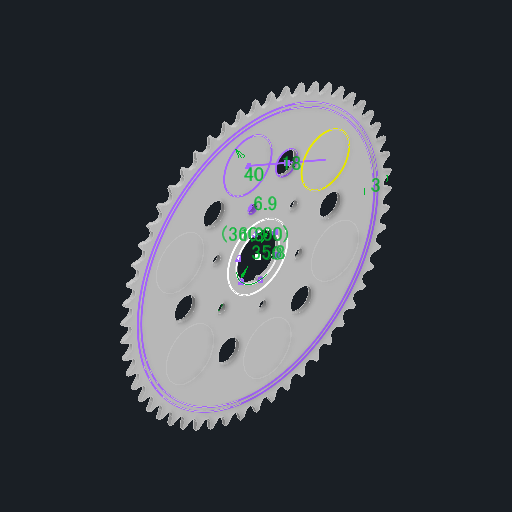
# Autodesk Inventor part: 410A54_()
Saved by Autodesk Inventor 2025.2 (Build 292293000, 293)
## iProperties
Category: PARTsolutions
Company: KANA
Created: 2025-03-16
Part Number: 410A54_()
Material: Generic
Catalog Web Link: www.cadenas.de
Description: 410A-Un-finished
Vendor: KANA
Document SubType Name: Modeling
Designer: psAdmin
Manufacturer: KANA
Mass: 102.167 g
Surface Area: 762.68 cm^2
Volume: 102.167 cm^3
Density: 1 g/cm^3
Appearance: PSOLRGB-175-175-175
PSOL_IDENT_0: {$CADENAS_DATA/23d-libs/kana/sprockets/chain_no_410/un_finished_sprocket_steel/a_type/410a.prj},159
PSOL_IDENT_1: {VTYP=3D},{NB=410A54_()},{LINA=410A54},{NN=410A},{DATE=27.06.2023 01:46:24},{GEOMDATE=02.10.2020 05:
PSOL_IDENT_2: 05:48},{VERSION=},{LINEID=690},{WBVAR=SURFT},{WBNUMERIC=}  {NB=410A54_()},{LINA=410A54},{KT=DUMMY},{
PSOL_IDENT_3: ORDERNO=410A54},{TYPE=410A},{NOT=54},{NOTX=54.000},{DP=218.42},{DC=210.67},{DC2=210.67},{DO=226},{T=
PSOL_IDENT_4: 2.8},{DR=7.750},{MAT=None},{MATC=},{SD=16},{SURFT=},{SURFTNB=},{DCX2=0},{CAUTION=The tooth profile i
PSOL_IDENT_5: n the CAD models differ from the actual shape.}
NB: 410A54_()
NN: 410A
NT: Un-finished
NBSYN: 410A$NOT._($SURFT.)
LINA: 410A54
CATALOG: KANA
TYPE: 410A
NOT: 54
DP: 218.42
DC: 210.67
DC2: 210.67
DO: 226
T: 2.8
SD: 16
SURFT: No symbol : No
CAUTION: The tooth profile in the CAD models differ from the actual shape.
SUPPLIER: KANA
ARTICLENO: 410A54_()
BOMINFO: 410A54
CREATOR: CADENAS GmbH
Title: 410A54
Author: Cadenas PARTsolutions
Comments: Un-finished
Autodesk Inventor part; units mm, degrees
sketch "Sketch_1" plane through (0, 0, 0) normal (0, 0, 1) x (1, 0, 0)
  line L0 (2.8, 0) -> (0, 0)
  line L1 (0, 8) -> (2.8, 8)
  line L2 (2.8, 8) -> (2.8, 111.7584)
  arc A0 (2.8, 111.7584) -> (2.1, 113) centre (-4.2724, 108.5892) ccw
  line L3 (2.1, 113) -> (0.7, 113)
  arc A1 (0.7, 113) -> (0, 111.7584) centre (7.0724, 108.5892) ccw
  line L4 (0, 111.7584) -> (0, 8)
  constraints: 10 end point, 4 point on circle, 2 centre point
revolve "Revolution1" add sketch "Sketch_1" angle 360 about axis through (2.8, 0, 0) along (1, 0, 0)
sketch "Sketch_2" plane through (1.4, 0, 0) normal (1, 0, 0) x (0, 0, -1)
  circle A0 centre (0, 0) radius 150.6667
  line L0 (-112.8368, 6.0711) -> (-107.5161, 3.4852)
  arc A1 (-107.5161, -3.4852) -> (-107.5161, 3.4852) centre (-109.21, 0) ccw
  line L1 (-107.5161, -3.4852) -> (-112.8368, -6.0711)
  arc A2 (-112.8368, -6.0711) -> (-112.7786, -7.0695) centre (0, 0) ccw
  line L2 (-112.7786, -7.0695) -> (-107.1937, -9.0203)
  arc A3 (-106.3845, -15.9435) -> (-107.1937, -9.0203) centre (-108.4716, -12.6785) ccw
  line L3 (-106.3845, -15.9435) -> (-111.369, -19.1296)
  arc A4 (-111.369, -19.1296) -> (-111.1954, -20.1145) centre (0, 0) ccw
  line L4 (-111.1954, -20.1145) -> (-105.4217, -21.4037)
  arc A5 (-103.8143, -28.1861) -> (-105.4217, -21.4037) centre (-106.2662, -25.1856) ccw
  line L5 (-103.8143, -28.1861) -> (-108.3952, -31.9295)
  arc A6 (-108.3952, -31.9295) -> (-108.1084, -32.8874) centre (0, 0) ccw
  line L6 (-108.1084, -32.8874) -> (-102.2241, -33.4977)
  arc A7 (-99.8401, -40.0477) -> (-102.2241, -33.4977) centre (-102.6238, -37.352) ccw
  line L7 (-99.8401, -40.0477) -> (-103.9554, -44.2975)
  arc A8 (-103.9554, -44.2975) -> (-103.5594, -45.2157) centre (0, 0) ccw
  line L8 (-103.5594, -45.2157) -> (-97.6441, -45.1387)
  arc A9 (-94.5158, -51.3676) -> (-97.6441, -45.1387) centre (-97.5936, -49.0134) ccw
  line L9 (-94.5158, -51.3676) -> (-98.1099, -56.0664)
  arc A10 (-98.1099, -56.0664) -> (-97.6099, -56.9325) centre (0, 0) ccw
  line L10 (-97.6099, -56.9325) -> (-91.7435, -56.1693)
  arc A11 (-87.9133, -61.9929) -> (-91.7435, -56.1693) centre (-91.2436, -60.0119) ccw
  line L11 (-87.9133, -61.9929) -> (-90.9376, -67.0772)
  arc A12 (-90.9376, -67.0772) -> (-90.3405, -67.8793) centre (0, 0) ccw
  line L12 (-90.3405, -67.8793) -> (-84.6023, -66.4402)
  arc A13 (-80.1219, -71.7798) -> (-84.6023, -66.4402) centre (-83.6597, -70.1988) ccw
  line L13 (-80.1219, -71.7798) -> (-82.5355, -77.1809)
  arc A14 (-82.5355, -77.1809) -> (-81.8493, -77.9082) centre (0, 0) ccw
  line L14 (-81.8493, -77.9082) -> (-76.3171, -75.8127)
  arc A15 (-71.247, -80.5961) -> (-76.3171, -75.8127) centre (-74.9444, -79.4365) ccw
  line L15 (-71.247, -80.5961) -> (-73.0173, -86.2408)
  arc A16 (-73.0173, -86.2408) -> (-72.2513, -86.8836) centre (0, 0) ccw
  line L16 (-72.2513, -86.8836) -> (-66.9997, -84.16)
  arc A17 (-61.4086, -88.3224) -> (-66.9997, -84.16) centre (-65.2157, -87.5999) ccw
  line L17 (-61.4086, -88.3224) -> (-62.5117, -94.1344)
  arc A18 (-62.5117, -94.1344) -> (-61.6762, -94.684) centre (0, 0) ccw
  line L18 (-61.6762, -94.684) -> (-56.7763, -91.3691)
  arc A19 (-50.7398, -94.8543) -> (-56.7763, -91.3691) centre (-54.605, -94.5786) ccw
  line L19 (-50.7398, -94.8543) -> (-51.1606, -100.7551)
  arc A20 (-51.1606, -100.7551) -> (-50.267, -101.2039) centre (0, 0) ccw
  line L20 (-50.267, -101.2039) -> (-45.7851, -97.3426)
  arc A21 (-39.3848, -100.1034) -> (-45.7851, -97.3426) centre (-43.2559, -100.2784) ccw
  line L21 (-39.3848, -100.1034) -> (-39.1177, -106.0132)
  arc A22 (-39.1177, -106.0132) -> (-38.1781, -106.3552) centre (0, 0) ccw
  line L22 (-38.1781, -106.3552) -> (-34.1747, -101.9998)
  arc A23 (-27.4972, -103.9989) -> (-34.1747, -101.9998) centre (-31.3218, -104.622) ccw
  line L23 (-27.4972, -103.9989) -> (-26.5459, -109.8377)
  arc A24 (-26.5459, -109.8377) -> (-25.5728, -110.0683) centre (0, 0) ccw
  line L24 (-25.5728, -110.0683) -> (-22.1022, -105.2775)
  arc A25 (-15.2378, -106.4879) -> (-22.1022, -105.2775) centre (-18.9641, -107.5509) ccw
  line L25 (-15.2378, -106.4879) -> (-13.615, -112.1768)
  arc A26 (-13.615, -112.1768) -> (-12.6218, -112.2929) centre (0, 0) ccw
  line L26 (-12.6218, -112.2929) -> (-9.7308, -107.1316)
  arc A27 (-2.7722, -107.5369) -> (-9.7308, -107.1316) centre (-6.35, -109.0252) ccw
  line L27 (-2.7722, -107.5369) -> (-0.5, -112.9989)
  arc A28 (-0.5, -112.9989) -> (0.5, -112.9989) centre (0, 0) ccw
  line L28 (0.5, -112.9989) -> (2.7722, -107.5369)
  arc A29 (9.7308, -107.1316) -> (2.7722, -107.5369) centre (6.35, -109.0252) ccw
  line L29 (9.7308, -107.1316) -> (12.6218, -112.2929)
  arc A30 (12.6218, -112.2929) -> (13.615, -112.1768) centre (0, 0) ccw
  line L30 (13.615, -112.1768) -> (15.2378, -106.4879)
  arc A31 (22.1022, -105.2775) -> (15.2378, -106.4879) centre (18.9641, -107.5509) ccw
  line L31 (22.1022, -105.2775) -> (25.5728, -110.0683)
  arc A32 (25.5728, -110.0683) -> (26.5459, -109.8377) centre (0, 0) ccw
  line L32 (26.5459, -109.8377) -> (27.4972, -103.9989)
  arc A33 (34.1747, -101.9998) -> (27.4972, -103.9989) centre (31.3218, -104.622) ccw
  line L33 (34.1747, -101.9998) -> (38.1781, -106.3552)
  arc A34 (38.1781, -106.3552) -> (39.1177, -106.0132) centre (0, 0) ccw
  line L34 (39.1177, -106.0132) -> (39.3848, -100.1034)
  arc A35 (45.7851, -97.3426) -> (39.3848, -100.1034) centre (43.2559, -100.2784) ccw
  line L35 (45.7851, -97.3426) -> (50.267, -101.2039)
  arc A36 (50.267, -101.2039) -> (51.1606, -100.7551) centre (0, 0) ccw
  line L36 (51.1606, -100.7551) -> (50.7398, -94.8543)
  arc A37 (56.7763, -91.3691) -> (50.7398, -94.8543) centre (54.605, -94.5786) ccw
  line L37 (56.7763, -91.3691) -> (61.6762, -94.684)
  arc A38 (61.6762, -94.684) -> (62.5117, -94.1344) centre (0, 0) ccw
  line L38 (62.5117, -94.1344) -> (61.4086, -88.3224)
  arc A39 (66.9997, -84.16) -> (61.4086, -88.3224) centre (65.2157, -87.5999) ccw
  line L39 (66.9997, -84.16) -> (72.2513, -86.8836)
  arc A40 (72.2513, -86.8836) -> (73.0173, -86.2408) centre (0, 0) ccw
  line L40 (73.0173, -86.2408) -> (71.247, -80.5961)
  arc A41 (76.3171, -75.8127) -> (71.247, -80.5961) centre (74.9444, -79.4365) ccw
  line L41 (76.3171, -75.8127) -> (81.8493, -77.9082)
  arc A42 (81.8493, -77.9082) -> (82.5355, -77.1809) centre (0, 0) ccw
  line L42 (82.5355, -77.1809) -> (80.1219, -71.7798)
  arc A43 (84.6023, -66.4402) -> (80.1219, -71.7798) centre (83.6597, -70.1988) ccw
  line L43 (84.6023, -66.4402) -> (90.3405, -67.8793)
  arc A44 (90.3405, -67.8793) -> (90.9376, -67.0772) centre (0, 0) ccw
  line L44 (90.9376, -67.0772) -> (87.9133, -61.9929)
  arc A45 (91.7435, -56.1693) -> (87.9133, -61.9929) centre (91.2436, -60.0119) ccw
  line L45 (91.7435, -56.1693) -> (97.6099, -56.9325)
  arc A46 (97.6099, -56.9325) -> (98.1099, -56.0664) centre (0, 0) ccw
  line L46 (98.1099, -56.0664) -> (94.5158, -51.3676)
  arc A47 (97.6441, -45.1387) -> (94.5158, -51.3676) centre (97.5936, -49.0134) ccw
  line L47 (97.6441, -45.1387) -> (103.5594, -45.2157)
  arc A48 (103.5594, -45.2157) -> (103.9554, -44.2975) centre (0, 0) ccw
  line L48 (103.9554, -44.2975) -> (99.8401, -40.0477)
  arc A49 (102.2241, -33.4977) -> (99.8401, -40.0477) centre (102.6238, -37.352) ccw
  line L49 (102.2241, -33.4977) -> (108.1084, -32.8874)
  arc A50 (108.1084, -32.8874) -> (108.3952, -31.9295) centre (0, 0) ccw
  line L50 (108.3952, -31.9295) -> (103.8143, -28.1861)
  arc A51 (105.4217, -21.4037) -> (103.8143, -28.1861) centre (106.2662, -25.1856) ccw
  line L51 (105.4217, -21.4037) -> (111.1954, -20.1145)
  arc A52 (111.1954, -20.1145) -> (111.369, -19.1296) centre (0, 0) ccw
  line L52 (111.369, -19.1296) -> (106.3845, -15.9435)
  arc A53 (107.1937, -9.0203) -> (106.3845, -15.9435) centre (108.4716, -12.6785) ccw
  line L53 (107.1937, -9.0203) -> (112.7786, -7.0695)
  arc A54 (112.7786, -7.0695) -> (112.8368, -6.0711) centre (0, 0) ccw
  line L54 (112.8368, -6.0711) -> (107.5161, -3.4852)
  arc A55 (107.5161, 3.4852) -> (107.5161, -3.4852) centre (109.21, 0) ccw
  line L55 (107.5161, 3.4852) -> (112.8368, 6.0711)
  arc A56 (112.8368, 6.0711) -> (112.7786, 7.0695) centre (0, 0) ccw
  line L56 (112.7786, 7.0695) -> (107.1937, 9.0203)
  arc A57 (106.3845, 15.9435) -> (107.1937, 9.0203) centre (108.4716, 12.6785) ccw
  line L57 (106.3845, 15.9435) -> (111.369, 19.1296)
  arc A58 (111.369, 19.1296) -> (111.1954, 20.1145) centre (0, 0) ccw
  line L58 (111.1954, 20.1145) -> (105.4217, 21.4037)
  arc A59 (103.8143, 28.1861) -> (105.4217, 21.4037) centre (106.2662, 25.1856) ccw
  line L59 (103.8143, 28.1861) -> (108.3952, 31.9295)
  arc A60 (108.3952, 31.9295) -> (108.1084, 32.8874) centre (0, 0) ccw
  line L60 (108.1084, 32.8874) -> (102.2241, 33.4977)
  arc A61 (99.8401, 40.0477) -> (102.2241, 33.4977) centre (102.6238, 37.352) ccw
  line L61 (99.8401, 40.0477) -> (103.9554, 44.2975)
  arc A62 (103.9554, 44.2975) -> (103.5594, 45.2157) centre (0, 0) ccw
  line L62 (103.5594, 45.2157) -> (97.6441, 45.1387)
  arc A63 (94.5158, 51.3676) -> (97.6441, 45.1387) centre (97.5936, 49.0134) ccw
  line L63 (94.5158, 51.3676) -> (98.1099, 56.0664)
  arc A64 (98.1099, 56.0664) -> (97.6099, 56.9325) centre (0, 0) ccw
  line L64 (97.6099, 56.9325) -> (91.7435, 56.1693)
  arc A65 (87.9133, 61.9929) -> (91.7435, 56.1693) centre (91.2436, 60.0119) ccw
  line L65 (87.9133, 61.9929) -> (90.9376, 67.0772)
  arc A66 (90.9376, 67.0772) -> (90.3405, 67.8793) centre (0, 0) ccw
  line L66 (90.3405, 67.8793) -> (84.6023, 66.4402)
  arc A67 (80.1219, 71.7798) -> (84.6023, 66.4402) centre (83.6597, 70.1988) ccw
  line L67 (80.1219, 71.7798) -> (82.5355, 77.1809)
  arc A68 (82.5355, 77.1809) -> (81.8493, 77.9082) centre (0, 0) ccw
  line L68 (81.8493, 77.9082) -> (76.3171, 75.8127)
  arc A69 (71.247, 80.5961) -> (76.3171, 75.8127) centre (74.9444, 79.4365) ccw
  line L69 (71.247, 80.5961) -> (73.0173, 86.2408)
  arc A70 (73.0173, 86.2408) -> (72.2513, 86.8836) centre (0, 0) ccw
  line L70 (72.2513, 86.8836) -> (66.9997, 84.16)
  arc A71 (61.4086, 88.3224) -> (66.9997, 84.16) centre (65.2157, 87.5999) ccw
  line L71 (61.4086, 88.3224) -> (62.5117, 94.1344)
  arc A72 (62.5117, 94.1344) -> (61.6762, 94.684) centre (0, 0) ccw
  line L72 (61.6762, 94.684) -> (56.7763, 91.3691)
  arc A73 (50.7398, 94.8543) -> (56.7763, 91.3691) centre (54.605, 94.5786) ccw
  line L73 (50.7398, 94.8543) -> (51.1606, 100.7551)
  arc A74 (51.1606, 100.7551) -> (50.267, 101.2039) centre (0, 0) ccw
  line L74 (50.267, 101.2039) -> (45.7851, 97.3426)
  arc A75 (39.3848, 100.1034) -> (45.7851, 97.3426) centre (43.2559, 100.2784) ccw
  line L75 (39.3848, 100.1034) -> (39.1177, 106.0132)
  arc A76 (39.1177, 106.0132) -> (38.1781, 106.3552) centre (0, 0) ccw
  line L76 (38.1781, 106.3552) -> (34.1747, 101.9998)
  arc A77 (27.4972, 103.9989) -> (34.1747, 101.9998) centre (31.3218, 104.622) ccw
  line L77 (27.4972, 103.9989) -> (26.5459, 109.8377)
  arc A78 (26.5459, 109.8377) -> (25.5728, 110.0683) centre (0, 0) ccw
  line L78 (25.5728, 110.0683) -> (22.1022, 105.2775)
  arc A79 (15.2378, 106.4879) -> (22.1022, 105.2775) centre (18.9641, 107.5509) ccw
  line L79 (15.2378, 106.4879) -> (13.615, 112.1768)
  arc A80 (13.615, 112.1768) -> (12.6218, 112.2929) centre (0, 0) ccw
  line L80 (12.6218, 112.2929) -> (9.7308, 107.1316)
  arc A81 (2.7722, 107.5369) -> (9.7308, 107.1316) centre (6.35, 109.0252) ccw
  line L81 (2.7722, 107.5369) -> (0.5, 112.9989)
  arc A82 (0.5, 112.9989) -> (-0.5, 112.9989) centre (0, 0) ccw
  line L82 (-0.5, 112.9989) -> (-2.7722, 107.5369)
  arc A83 (-9.7308, 107.1316) -> (-2.7722, 107.5369) centre (-6.35, 109.0252) ccw
  line L83 (-9.7308, 107.1316) -> (-12.6218, 112.2929)
  arc A84 (-12.6218, 112.2929) -> (-13.615, 112.1768) centre (0, 0) ccw
  line L84 (-13.615, 112.1768) -> (-15.2378, 106.4879)
  arc A85 (-22.1022, 105.2775) -> (-15.2378, 106.4879) centre (-18.9641, 107.5509) ccw
  line L85 (-22.1022, 105.2775) -> (-25.5728, 110.0683)
  arc A86 (-25.5728, 110.0683) -> (-26.5459, 109.8377) centre (0, 0) ccw
  line L86 (-26.5459, 109.8377) -> (-27.4972, 103.9989)
  arc A87 (-34.1747, 101.9998) -> (-27.4972, 103.9989) centre (-31.3218, 104.622) ccw
  line L87 (-34.1747, 101.9998) -> (-38.1781, 106.3552)
  arc A88 (-38.1781, 106.3552) -> (-39.1177, 106.0132) centre (0, 0) ccw
  line L88 (-39.1177, 106.0132) -> (-39.3848, 100.1034)
  arc A89 (-45.7851, 97.3426) -> (-39.3848, 100.1034) centre (-43.2559, 100.2784) ccw
  line L89 (-45.7851, 97.3426) -> (-50.267, 101.2039)
  arc A90 (-50.267, 101.2039) -> (-51.1606, 100.7551) centre (0, 0) ccw
  line L90 (-51.1606, 100.7551) -> (-50.7398, 94.8543)
  arc A91 (-56.7763, 91.3691) -> (-50.7398, 94.8543) centre (-54.605, 94.5786) ccw
  line L91 (-56.7763, 91.3691) -> (-61.6762, 94.684)
  arc A92 (-61.6762, 94.684) -> (-62.5117, 94.1344) centre (0, 0) ccw
  line L92 (-62.5117, 94.1344) -> (-61.4086, 88.3224)
  arc A93 (-66.9997, 84.16) -> (-61.4086, 88.3224) centre (-65.2157, 87.5999) ccw
  line L93 (-66.9997, 84.16) -> (-72.2513, 86.8836)
  arc A94 (-72.2513, 86.8836) -> (-73.0173, 86.2408) centre (0, 0) ccw
  line L94 (-73.0173, 86.2408) -> (-71.247, 80.5961)
  arc A95 (-76.3171, 75.8127) -> (-71.247, 80.5961) centre (-74.9444, 79.4365) ccw
  line L95 (-76.3171, 75.8127) -> (-81.8493, 77.9082)
  arc A96 (-81.8493, 77.9082) -> (-82.5355, 77.1809) centre (0, 0) ccw
  line L96 (-82.5355, 77.1809) -> (-80.1219, 71.7798)
  arc A97 (-84.6023, 66.4402) -> (-80.1219, 71.7798) centre (-83.6597, 70.1988) ccw
  line L97 (-84.6023, 66.4402) -> (-90.3405, 67.8793)
  arc A98 (-90.3405, 67.8793) -> (-90.9376, 67.0772) centre (0, 0) ccw
  line L98 (-90.9376, 67.0772) -> (-87.9133, 61.9929)
  arc A99 (-91.7435, 56.1693) -> (-87.9133, 61.9929) centre (-91.2436, 60.0119) ccw
  line L99 (-91.7435, 56.1693) -> (-97.6099, 56.9325)
  arc A100 (-97.6099, 56.9325) -> (-98.1099, 56.0664) centre (0, 0) ccw
  line L100 (-98.1099, 56.0664) -> (-94.5158, 51.3676)
  arc A101 (-97.6441, 45.1387) -> (-94.5158, 51.3676) centre (-97.5936, 49.0134) ccw
  line L101 (-97.6441, 45.1387) -> (-103.5594, 45.2157)
  arc A102 (-103.5594, 45.2157) -> (-103.9554, 44.2975) centre (0, 0) ccw
  line L102 (-103.9554, 44.2975) -> (-99.8401, 40.0477)
  arc A103 (-102.2241, 33.4977) -> (-99.8401, 40.0477) centre (-102.6238, 37.352) ccw
  line L103 (-102.2241, 33.4977) -> (-108.1084, 32.8874)
  arc A104 (-108.1084, 32.8874) -> (-108.3952, 31.9295) centre (0, 0) ccw
  line L104 (-108.3952, 31.9295) -> (-103.8143, 28.1861)
  arc A105 (-105.4217, 21.4037) -> (-103.8143, 28.1861) centre (-106.2662, 25.1856) ccw
  line L105 (-105.4217, 21.4037) -> (-111.1954, 20.1145)
  arc A106 (-111.1954, 20.1145) -> (-111.369, 19.1296) centre (0, 0) ccw
  line L106 (-111.369, 19.1296) -> (-106.3845, 15.9435)
  arc A107 (-107.1937, 9.0203) -> (-106.3845, 15.9435) centre (-108.4716, 12.6785) ccw
  line L107 (-107.1937, 9.0203) -> (-112.7786, 7.0695)
  arc A108 (-112.7786, 7.0695) -> (-112.8368, 6.0711) centre (0, 0) ccw
  constraints: 216 end point, 216 point on circle, 109 centre point
extrude "Extrusion1" cut sketch "Sketch_2" along normal mid plane 3.2
ref_plane "Body_XY" through (0, 0, 0) normal (1, 0, 0) x (0, 0, -1)
ref_plane "Body_YZ" through (0, 0, 0) normal (0, 0, -1) x (0, 1, 0)
ref_plane "Body_ZX" through (0, 0, 0) normal (0, 1, 0) x (1, 0, 0)
sketch "スケッチ3" plane through (2.8, 12.6785, -108.4716) normal (1, 0, 0) x (0, 0.1160929, -0.9932384)
  circle A0 centre (-109.21, 0) radius 17.9
  line L0 (-109.21, 17.9) -> (-109.21, 16.1)
  arc A1 (-109.21, 16.1) -> (-107.4122, 17.8118) centre (-109.21, 17.9) ccw
  arc A2 (-111.0077, 17.8095) -> (-109.21, 16.1) centre (-109.21, 17.9) ccw
  arc A3 (-123.153, 8.05) -> (-123.7366, 10.4629) centre (-124.7119, 8.95) ccw
  arc A4 (-125.5323, 7.3479) -> (-123.153, 8.05) centre (-124.7119, 8.95) ccw
  arc A5 (-123.153, -8.05) -> (-125.5344, -7.3489) centre (-124.7119, -8.95) ccw
  arc A6 (-123.7346, -10.4616) -> (-123.153, -8.05) centre (-124.7119, -8.95) ccw
  arc A7 (-109.21, -16.1) -> (-111.0078, -17.8118) centre (-109.21, -17.9) ccw
  arc A8 (-107.4123, -17.8095) -> (-109.21, -16.1) centre (-109.21, -17.9) ccw
  arc A9 (-95.267, -8.05) -> (-94.6834, -10.4629) centre (-93.7081, -8.95) ccw
  arc A10 (-92.8877, -7.3479) -> (-95.267, -8.05) centre (-93.7081, -8.95) ccw
  arc A11 (-95.267, 8.05) -> (-92.8856, 7.3489) centre (-93.7081, 8.95) ccw
  arc A12 (-94.6854, 10.4616) -> (-95.267, 8.05) centre (-93.7081, 8.95) ccw
  circle A13 centre (-109.21, 0) radius 25
  point P0 (-94.6854, 10.4616)
  point P1 (-107.4123, 17.8095)
  point P2 (-123.7346, 10.4616)
  point P3 (-125.5323, 7.3479)
  point P4 (-125.5323, -7.3479)
  point P5 (-123.7346, -10.4616)
  point P6 (-111.0077, -17.8095)
  point P7 (-94.6854, -10.4616)
  point P8 (-92.8877, 7.3479)
  dimension "d5" = 35.8
  dimension "d6" = 1.8
  dimension "d9" = 360
  dimension "d13" = 50
  constraints: 32 point on circle, 14 centre point, 9 coincident, 2 end point, 1 vertical, 43 other
  measures "d5" diameter of A0
  measures "d6" distance of L0.start L0.end
  measures "d13" diameter of A13
extrude "押し出し2" cut sketch "スケッチ3" against normal blind 10 contours A2 A1 A0 A12 A11 A10 A9 A8 A7 A6 A5 A4 A3
extrude "押し出し3" cut sketch "スケッチ3" against normal blind 0.3 contours L0 A2 A0 | A0 A1 L0 | A3 A4 A0 | A0 A11 A12 | A5 A6 A0 | A0 A9 A10 | A7 A8 A0 | A13
sketch "スケッチ4" plane through (2.8, 12.6785, -108.4716) normal (1, 0, 0) x (0, 0.1160929, -0.9932384)
  circle A0 centre (-109.21, 70.7972) radius 20
  circle A1 centre (-109.21, 37.4404) radius 3.45
  point P0 (-109.21, 0)
  dimension "d16" = 40
  dimension "d22" = 6.9
  constraints: 2 centre point
  measures "d16" diameter of A0
  measures "d22" diameter of A1
extrude "押し出し4" cut sketch "スケッチ4" against normal blind 0.3 contours A0
pattern_circular "円形状パターン1" count 6 over 360 about axis through (2.8, 0, 0) along (-1, 0, 0) of "押し出し4"
extrude "押し出し5" cut sketch "スケッチ4" against normal through all contours A1
pattern_circular "円形状パターン2" count 6 over 360 about axis through (2.8, 0, 0) along (-1, 0, 0) of "押し出し5"
sketch "スケッチ5" plane through (2.8, 12.6785, -108.4716) normal (1, 0, 0) x (0, 0.1160929, -0.9932384)
  circle A0 centre (-47.8978, 35.3986) radius 20 projected
  line L0 (-109.21, 70.7498) -> (-47.8978, 35.3986)
  circle A1 centre (-78.5539, 53.0742) radius 9
  circle A2 centre (-109.21, 0) radius 100.682
  circle A3 centre (-109.21, 0) radius 97.682
  dimension "d28" = 18
  dimension "d34" = 3
  constraints: 3 centre point, 2 coincident, 2 end point, 1 midpoint
  measures "d28" diameter of A1
  measures "d34" radial gap between concentric circles of A2 A3
extrude "押し出し6" cut sketch "スケッチ5" against normal blind 10 contours A1 L0 | L0 A1
pattern_circular "円形状パターン3" count 6 over 360 about axis through (2.8, 0, 0) along (-1, 0, 0) of "押し出し6"
extrude "押し出し7" cut sketch "スケッチ5" against normal blind 1 contours A2
body "Solid1"
